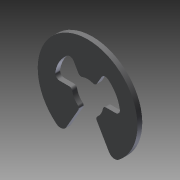
# Autodesk Inventor part: D-25369
Saved by Autodesk Inventor 2012 (Build 160160000, 160)
## iProperties
Created: 2013-01-17
Part Number: D-25369
Material: Default
Catalog Web Link: www.cadenas.de
Description: Piston Rod Clevis for Original Line Cylinders - Retaining Ring-
Vendor: BIMBA
Document SubType Name: Modeling
Designer: William
Manufacturer: BIMBA
Density: 1 g/cm^3
Category: PARTsolutions
Company: BIMBA
Title: D-25369
Author: Cadenas PARTsolutions
PSOL_IDENT_0: {\\10.0.0.242\data_v9\23d-libs\bimba\bimba\bimba_imperial\bimba_full_line\original_line_cylinders\ac
PSOL_IDENT_1: cessories\piston_rod_clevis_rr.prj},212 {VTYP=3D},{NB=D-25369},{LINA=D-25369},{NN=Piston Rod Clevis
PSOL_IDENT_2: for Original Line Cylinders - Retaining Ring},{DATE=06.12.2012 07:53:57},{GEOMDATE=06.12.2012 07:18:
PSOL_IDENT_3: 40},{VERSION=},{LINEID=10},{LINESUBID=-1},{WBVAR=}  {NB=D-25369},{LINA=D-25369},{KT=DUMMY},{PN=D-253
PSOL_IDENT_4: 69},{D=0.31000000},{D1=0.09650000},{D2=0.20325},{L=0.01500000},{COLOR=0.75,0.75,0.75,0.00}
CNS_NB: D-25369
CNS_NBSYN: $PN.
CNS_LINA: D-25369
CNS_PN: D-25369
CNS_D: 0.31000000
CNS_D1: 0.09650000
CNS_D2: 0.203
CNS_L: 0.01500000
CNS_COLOR: 0.75,0.75,0.75,0.00
SUPPLIER: BIMBA
ARTICLENO: D-25369
BOMINFO: D-25369
CREATOR: CADENAS GmbH
Autodesk Inventor part; units mm, degrees
sketch "Sketch_1" plane through (0, 0, 0) normal (0, 0, 1) x (1, 0, 0)
  arc A0 (2.4605, -3.0734) -> (-2.4605, -3.0734) centre (0, 0) ccw
  arc A1 (-2.4605, -3.0734) -> (-1.6908, -2.9285) centre (-2.1379, -2.6704) ccw
  line L0 (-1.6908, -2.9285) -> (-0.725, -1.2558)
  arc A2 (-0.725, -1.2558) -> (-0.7811, -0.9444) centre (-0.9373, -1.1333) ccw
  arc A3 (-1.2084, -0.2043) -> (-0.7811, -0.9444) centre (0, 0) ccw
  arc A4 (-1.2084, -0.2043) -> (-1.4501, 0) centre (-1.4501, -0.2451) ccw
  line L1 (-1.4501, 0) -> (-2.2105, 0)
  arc A5 (-2.5505, 0.3971) -> (-2.2105, 0) centre (-2.2105, 0.3442) ccw
  arc A6 (-1.6192, 2.0103) -> (-2.5505, 0.3971) centre (0, 0) ccw
  arc A7 (-1.1052, 1.9143) -> (-1.6192, 2.0103) centre (-1.4033, 1.7422) ccw
  line L2 (-1.1052, 1.9143) -> (-0.725, 1.2558)
  arc A8 (-0.725, 1.2558) -> (-0.4273, 1.1486) centre (-0.5128, 1.3784) ccw
  arc A9 (0.4273, 1.1486) -> (-0.4273, 1.1486) centre (0, 0) ccw
  arc A10 (0.4273, 1.1486) -> (0.725, 1.2558) centre (0.5128, 1.3784) ccw
  line L3 (0.725, 1.2558) -> (1.1052, 1.9143)
  arc A11 (1.6192, 2.0103) -> (1.1052, 1.9143) centre (1.4033, 1.7422) ccw
  arc A12 (2.5505, 0.3971) -> (1.6192, 2.0103) centre (0, 0) ccw
  arc A13 (2.2105, 0) -> (2.5505, 0.3971) centre (2.2105, 0.3442) ccw
  line L4 (2.2105, 0) -> (1.4501, 0)
  arc A14 (1.4501, 0) -> (1.2084, -0.2043) centre (1.4501, -0.2451) ccw
  arc A15 (0.7811, -0.9444) -> (1.2084, -0.2043) centre (0, 0) ccw
  arc A16 (0.7811, -0.9444) -> (0.725, -1.2558) centre (0.9373, -1.1333) ccw
  line L5 (0.725, -1.2558) -> (1.6908, -2.9285)
  arc A17 (1.6908, -2.9285) -> (2.4605, -3.0734) centre (2.1379, -2.6704) ccw
  constraints: 36 point on circle, 18 centre point, 12 end point
extrude "Extrusion1" add sketch "Sketch_1" along normal mid plane 0.381
ref_plane "RR_XY" through (0, 0, 0) normal (0, 0, 1) x (1, 0, 0)
ref_plane "RR_YZ" through (0, 0, 0) normal (1, 0, 0) x (0, 1, 0)
ref_plane "RR_ZX" through (0, 0, 0) normal (0, 1, 0) x (0, 0, 1)
body "Solid1"
